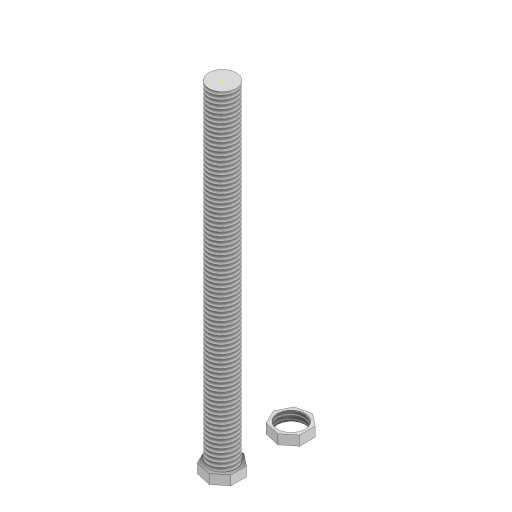
# Autodesk Inventor part: torniquete feo
Saved by Autodesk Inventor 2024.3 (Build 283343000, 343)
## iProperties
Created: 2025-09-23
Part Number: torniquete feo
Material: Generic
Document SubType Name: Modeling
Designer: danie
Density: 1 g/cm^3
Appearance: Default
Author: danie
Autodesk Inventor part; units mm, degrees
ref_plane "YZ Plane" through (0, 0, 0) normal (1, 0, 0) x (0, 1, 0)
ref_plane "XZ Plane" through (0, 0, 0) normal (0, 1, 0) x (-1, 0, 0)
ref_plane "XY Plane" through (0, 0, 0) normal (0, 0, 1) x (1, 0, 0)
sketch "Sketch1" plane through (0, 0, 0) normal (0, 1, 0) x (-1, 0, 0)
  circle A0 centre (0, 0) radius 4.375
  line L0 (4.375, 0) -> (2.7278, -3.4205)
  line L1 (2.7278, -3.4205) -> (-0.9735, -4.2653)
  line L2 (-0.9735, -4.2653) -> (-3.9417, -1.8982)
  line L3 (-3.9417, -1.8982) -> (-3.9417, 1.8982)
  line L4 (-3.9417, 1.8982) -> (-0.9735, 4.2653)
  line L5 (-0.9735, 4.2653) -> (2.7278, 3.4205)
  line L6 (2.7278, 3.4205) -> (4.375, 0)
  dimension "d0" = 8.75
  constraints: 14 end point, 2 coincident, 1 horizontal alignment, 17 other
extrude "Extrusion1" add sketch "Sketch1" along normal blind 2.35 contours L0 L1 L2 L3 L4 L5 L6
sketch "Sketch2" plane through (0, 2.35, 0) normal (0, 1, 0) x (1, 0, 0)
  circle A0 centre (0, 0) radius 3.375
  dimension "d3" = 6.75
  constraints: 1 centre point, 1 coincident
  measures "d3" diameter of A0
extrude "Extrusion2" add sketch "Sketch2" along normal blind 80.751
thread "Thread1" size "M7x1" class "6g" standard "ANSI Metric M Profile" full length
sketch "Sketch3" plane through (0, 83.101, 0) normal (0, 1, 0) x (1, 0, 0)
  point P0 (0, 0)
sketch "Sketch4" plane through (0, 0, 0) normal (0, -1, 0) x (1, 0, 0)
  circle A0 centre (0, -16.8413) radius 4.375
  line L0 (-4.375, -16.8413) -> (-2.7278, -13.4208)
  line L1 (-2.7278, -13.4208) -> (0.9735, -12.576)
  line L2 (0.9735, -12.576) -> (3.9417, -14.943)
  line L3 (3.9417, -14.943) -> (3.9417, -18.7395)
  line L4 (3.9417, -18.7395) -> (0.9735, -21.1066)
  line L5 (0.9735, -21.1066) -> (-2.7278, -20.2618)
  line L6 (-2.7278, -20.2618) -> (-4.375, -16.8413)
  point P0 (0, 0)
  dimension "d8" = 8.75
  constraints: 14 end point, 1 coincident, 1 horizontal alignment, 17 other
sketch "Sketch5" plane through (-4.375, 0, 0) normal (-0.9009689, 0, -0.4338837) x (-0.4338837, 0, 0.9009689)
  point P0 (-1.8982, 0)
extrude "Extrusion3" add sketch "Sketch4" against normal blind 2.35 contours L3 L4 L5 L6 L0 L1 L2
sketch "Sketch6" plane through (0, 83.101, 0) normal (0, 1, 0) x (1, 0, 0)
  point P0 (0, 0)
sketch "Sketch7" plane through (0, 2.35, 0) normal (0, 1, 0) x (1, 0, 0)
  line L0 (3.9417, 14.943) -> (3.9417, 18.7395) projected
  line L1 (3.9417, 14.943) -> (3.9417, 16.841)
  line L2 (-2.7278, 20.2618) -> (-4.375, 16.8413) projected
  line L3 (3.9417, 16.841) -> (-4.375, 16.8413)
  line L4 (3.9417, 14.943) -> (2.4576, 13.7595)
  line L5 (2.4576, 13.7595) -> (-2.7278, 20.2618)
  circle A0 centre (0.0001, 16.8411) radius 3.375
  point P0 (0, 0)
  dimension "d11" = 1.898
  dimension "d12" = 6.75
  constraints: 8 end point, 3 point on line, 1 centre point, 1 perpendicular
  measures "d11" distance of L0.start L1.end
  measures "d12" diameter of A0
extrude "Extrusion4" cut sketch "Sketch7" against normal blind 2.35 contours A0 L5 L3 | L3 L5 A0 | A0 L3 L5 | L3 A0 L5
thread "Thread2" size "M7x1" class "6H" standard "ANSI Metric M Profile" full length
body "Solid1"
